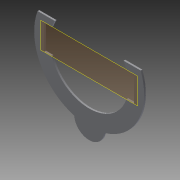
# Autodesk Inventor part: gyroYoke01
Saved by Autodesk Inventor 2013 (Build 170138000, 138)
## iProperties
Created: 2013-02-24
Part Number: gyroYoke01
Material: Generic
Document SubType Name: Modeling
Designer: Nano
Density: 1 g/cm^3
d0: 0.125 in
d1: 1.000 in
d3: 0.250 in
d4: 0.00 deg
d5: 0.250 in
d6: 0.250 in
d7: 0.250 in
d8: 0.250 in
Author: Nano
Autodesk Inventor part; units mm, degrees
ref_plane "YZ Plane" through (0, 0, 0) normal (1, 0, 0) x (0, 1, 0)
ref_plane "XZ Plane" through (0, 0, 0) normal (0, 1, 0) x (-1, 0, 0)
ref_plane "XY Plane" through (0, 0, 0) normal (0, 0, 1) x (1, 0, 0)
ref_plane "Work Plane1" through (0, 0, 0) normal (0, 0, 1) x (1, 0, 0)
sketch "Sketch1" plane through (0, 0, 0) normal (0, 0, 1) x (1, 0, 0)
  circle A0 centre (166.6875, 44.45) radius 6.35 construction
  line L0 (0, 0) -> (333.375, 0) construction
  line L1 (333.375, 0) -> (333.375, 88.9) construction
  line L2 (0, 88.9) -> (333.375, 88.9) construction
  line L3 (0, 0) -> (0, 88.9) construction
  line L4 (336.55, 95.25) -> (336.55, -6.35)
  line L5 (-3.175, -6.35) -> (-3.175, 95.25)
  arc A1 (361.952, -28.5758) -> (361.6406, 118.3031) centre (166.6875, 44.45) ccw
  arc A2 (109.447, -157.0949) -> (223.6431, -156.0919) centre (166.5241, -154.21) ccw
  arc A3 (136.5157, -103.6516) -> (194.8252, -103.6516) centre (165.6705, 44.881) ccw
  arc A4 (223.6431, -156.0919) -> (361.952, -28.5758) centre (166.6875, 44.45) ccw
  arc A5 (-29.5537, -28.941) -> (109.447, -157.0949) centre (166.6875, 44.45) ccw
  arc A6 (-29.5402, 117.8769) -> (-29.5537, -28.941) centre (166.6875, 44.45) ccw
  arc A7 (336.55, 165.3087) -> (333.375, 169.6513) centre (166.6875, 44.45) ccw
  arc A8 (0, 169.6513) -> (-3.175, 165.3087) centre (166.6875, 44.45) ccw
  line L6 (361.6406, 118.3031) -> (296.5092, 118.3031)
  line L7 (35.5911, 117.8769) -> (-29.5402, 117.8769)
  arc A9 (194.8252, -103.6516) -> (308.104, -6.35) centre (165.6705, 44.881) ccw
  arc A10 (306.9947, 95.25) -> (296.5092, 118.3031) centre (165.6705, 44.881) ccw
  arc A11 (35.5911, 117.8769) -> (25.271, 95.25) centre (165.6705, 44.881) ccw
  arc A12 (23.237, -6.35) -> (136.5157, -103.6516) centre (165.6705, 44.881) ccw
  line L8 (-3.175, 95.25) -> (25.271, 95.25)
  line L9 (306.9947, 95.25) -> (336.55, 95.25)
  line L10 (336.55, -6.35) -> (308.104, -6.35)
  line L11 (23.237, -6.35) -> (-3.175, -6.35)
  dimension "d0" = 3.175
  dimension "d5" = 6.35
  dimension "d6" = 6.35
  dimension "d7" = 6.35
  dimension "d8" = 6.35
  constraints: 24 point on circle, 16 end point, 12 centre point, 4 point on line
  measures "d0" distance between parallel lines of L4 L1
  measures "d5" distance between parallel lines of L2 L9
  measures "d6" distance between parallel lines of L0 L10
  measures "d7" distance between parallel lines of L2 L8
  measures "d8" distance between parallel lines of L0 L11
extrude "Extrusion1" add sketch "Sketch1" against normal blind 6.35
equation "\"d6\" = d5"
equation "\"d7\" = d5"
equation "\"d8\" = d5"
body "Solid1"
